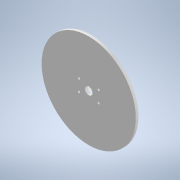
# Autodesk Inventor part: Base2
Saved by Autodesk Inventor 2021 (Build 250183000, 183)
## iProperties
Created: 2021-03-29
Part Number: Base2
Material: Genérico
Document SubType Name: Modeling
Designer: diego
Density: 1 g/cm^3
Appearance: Valor por defecto
Author: diego
Autodesk Inventor part; units mm, degrees
ref_plane "YZ Plane" through (0, 0, 0) normal (1, 0, 0) x (0, 1, 0)
ref_plane "XZ Plane" through (0, 0, 0) normal (0, 1, 0) x (-1, 0, 0)
ref_plane "XY Plane" through (0, 0, 0) normal (0, 0, 1) x (1, 0, 0)
sketch "Boceto1" plane through (0, 0, 0) normal (0, 0, 1) x (1, 0, 0)
  circle A0 centre (0, 0) radius 55
  constraints: 1 centre point, 1 coincident
extrude "Extrusión1" add sketch "Boceto1" against normal blind 3
sketch "Boceto2" plane through (0, 0, 0) normal (0, 0, 1) x (1, 0, 0)
  circle A0 centre (0, 0) radius 4.5
  constraints: 1 centre point, 1 coincident
hole "Agujero1" at (0, 0, 0) direction (0, 0, -1) diameter 9 end through all
sketch "Boceto3" plane through (0, 0, 0) normal (0, 0, 1) x (1, 0, 0)
  line L0 (0, 0) -> (-11.5, 0)
  circle A0 centre (-11.5, 6.75) radius 1.25
  circle A1 centre (11.5, 6.75) radius 1.25
  circle A2 centre (11.5, -6.75) radius 1.25
  circle A3 centre (-11.5, -6.75) radius 1.25
  constraints: 4 centre point, 2 end point, 1 horizontal
hole "Agujero2" at (11.5, -6.75, 0) at (-11.5, 6.75, 0) at (-11.5, -6.75, 0) at (11.5, 6.75, 0) direction (0, 0, -1) diameter 2.5 end through all
sketch "Boceto4" plane through (0, 0, -3) normal (0, 0, -1) x (-1, 0, 0)
  point P0 (0, 0)
